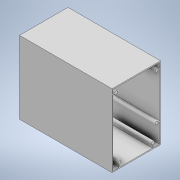
# Autodesk Inventor part: shell
Saved by Autodesk Inventor 2020.3 (Build 243373000, 373)
## iProperties
Created: 2020-08-10
Part Number: shell
Material: Generic
Document SubType Name: Modeling
Designer: joesp
Density: 1 g/cm^3
Appearance: Default
Author: joesp
Autodesk Inventor part; units mm, degrees
ref_plane "YZ Plane" through (0, 0, 0) normal (1, 0, 0) x (0, 1, 0)
ref_plane "XZ Plane" through (0, 0, 0) normal (0, 1, 0) x (-1, 0, 0)
ref_plane "XY Plane" through (0, 0, 0) normal (0, 0, 1) x (1, 0, 0)
sketch "Sketch1" plane through (0, 0, 0) normal (1, 0, 0) x (0, 1, 0)
  line L0 (0, 0) -> (147, 0)
  line L1 (147, 0) -> (147, 98)
  line L2 (147, 98) -> (0, 98)
  line L3 (0, 98) -> (0, 0)
  line L4 (2, 2) -> (145, 2)
  line L5 (145, 2) -> (145, 96)
  line L6 (145, 96) -> (2, 96)
  line L7 (2, 96) -> (2, 2)
  line L8 (137, 96) -> (135, 96)
  line L9 (135, 96) -> (135, 93)
  line L10 (135, 93) -> (137, 93)
  line L11 (137, 93) -> (137, 96)
  circle A0 centre (136, 90.1716) radius 3
  line L12 (135, 2) -> (133, 2)
  line L13 (133, 2) -> (133, 5)
  line L14 (133, 5) -> (135, 5)
  line L15 (135, 5) -> (135, 2)
  circle A1 centre (134, 7.8284) radius 3
  line L16 (2, 84) -> (8, 84)
  line L17 (8, 84) -> (8, 82)
  line L18 (8, 82) -> (2, 82)
  line L19 (2, 82) -> (2, 84)
  line L20 (2, 14) -> (8, 14)
  line L21 (8, 14) -> (8, 16)
  line L22 (8, 16) -> (2, 16)
  line L23 (2, 16) -> (2, 14)
  line L24 (41, 2) -> (43, 2)
  line L25 (43, 2) -> (43, 5)
  line L26 (43, 5) -> (41, 5)
  line L27 (41, 5) -> (41, 2)
  circle A2 centre (10.8284, 83) radius 3
  circle A3 centre (10.8284, 15) radius 3
  circle A4 centre (42, 7.8284) radius 3
  point P0 (2, 16)
  dimension "d36" = 2
  dimension "d37" = 2
  dimension "d38" = 2
  dimension "d39" = 2
  dimension "d40" = 98
  dimension "d41" = 147
  dimension "d42" = 2
  dimension "d43" = 3
  dimension "d44" = 6
  dimension "d45" = 11
  dimension "d46" = 3
  dimension "d47" = 2
  dimension "d48" = 6
  dimension "d49" = 11
  dimension "d50" = 2
  dimension "d51" = 2
  dimension "d52" = 6
  dimension "d53" = 2
  dimension "d54" = 3
  dimension "d55" = 6
  dimension "d56" = 6
  dimension "d57" = 6
  dimension "d58" = 15
  dimension "d60" = 15
  dimension "d61" = 42
  constraints: 56 end point, 14 parallel, 10 point on circle, 7 horizontal, 7 perpendicular, 6 point on line, 5 centre point, 1 coincident
  measures "d36" distance between parallel lines of L1 L5
  measures "d37" distance between parallel lines of L2 L6
  measures "d38" distance between parallel lines of L0 L4
  measures "d39" distance between parallel lines of L7 L3
  measures "d40" distance between parallel lines of L0 L2
  measures "d41" distance between parallel lines of L1 L3
  measures "d42" distance between parallel lines of L11 L9
  measures "d43" distance of L10.end L8.start
  measures "d44" diameter of A0
  measures "d45" distance from line of L1 A0.centre
  measures "d46" distance of L14.end L12.start
  measures "d47" distance of L13.end L14.end
  measures "d48" diameter of A1
  measures "d49" distance from line of L5 A1.centre
  measures "d50" distance of L16.end L17.end
  measures "d51" distance of L20.end L21.end
  measures "d52" distance of L17.end L18.end
  measures "d53" distance of L25.end L26.end
  measures "d54" distance of L24.end L25.end
  measures "d55" diameter of A2
  measures "d56" diameter of A3
  measures "d57" diameter of A4
  measures "d58" distance from line of L2 A2.centre
  measures "d60" distance from line of L0 A3.centre
  measures "d61" distance from line of L3 A4.centre
extrude "Extrusion1" add sketch "Sketch1" along normal blind 187 contours L3 L2 L1 L0 | L27 A4 L25 L4 | L7 L22 A3 L20 | A4 L26 | L26 A4 | A3 L21 | L21 A3 | L13 A1 L15 L4 | L7 L16 A2 L18 | A1 L14 | L14 A1 | A2 L17 | L17 A2 | L6 L11 A0 L9 | A0 L10 | L10 A0
equation "\"d37\" = d36"
equation "\"d38\" = d36"
equation "\"d39\" = d36"
equation "\"d46\" = d43"
equation "\"d47\" = d42"
equation "\"d48\" = d44"
equation "\"d49\" = d45"
equation "\"d50\" = d42"
equation "\"d51\" = d42"
equation "\"d53\" = d42"
equation "\"d54\" = d43"
equation "\"d55\" = d44"
equation "\"d56\" = d44"
equation "\"d57\" = d44"
body "Solid1"
